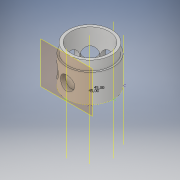
# Autodesk Inventor part: nozzle
Saved by Autodesk Inventor 2019 (Build 230136000, 136)
## iProperties
Created: 2020-10-28
Part Number: nozzle
Material: Genérico
Document SubType Name: Modeling
Designer: Juan M. Casillas
Density: 1 g/cm^3
Appearance: Valor por defecto
Author: Juan M. Casillas
## iProperties of the stored document nozzle_3DPrint.ipt
Created: 2020-10-28
Part Number: nozzle_3DPrint
Material: Genérico
Document SubType Name: Modeling
Designer: Juan M. Casillas
Density: 1 g/cm^3
Appearance: Valor por defecto
Author: Juan M. Casillas
Autodesk Inventor part; units mm, degrees
ref_plane "YZ Plane" through (0, 0, 0) normal (1, 0, 0) x (0, 1, 0)
ref_plane "XZ Plane" through (0, 0, 0) normal (0, 1, 0) x (-1, 0, 0)
ref_plane "XY Plane" through (0, 0, 0) normal (0, 0, 1) x (1, 0, 0)
sketch "Sketch1" plane through (0, 0, 0) normal (0, 1, 0) x (-1, 0, 0)
  circle A0 centre (0, 0) radius 4.65
  circle A1 centre (0, 0) radius 4.05
  dimension "d0" = 9.3
  dimension "d1" = 0.6
  constraints: 2 centre point, 1 coincident
  measures "d0" diameter of A0
  measures "d1" radial gap between concentric circles of A0 A1
extrude "Extrusion1" add sketch "Sketch1" along normal blind 2
sketch "Sketch2" plane through (0, 0, 0) normal (0, -1, 0) x (1, 0, 0)
  circle A0 centre (0, 0) radius 5
  dimension "d4" = 10
  constraints: 1 centre point, 1 coincident
  measures "d4" diameter of A0
extrude "Extrusion2" add sketch "Sketch2" along normal blind 5
sketch "Sketch3" plane through (0, 0, 0) normal (0, 1, 0) x (1, 0, 0)
  circle A0 centre (0, 0) radius 4.05 projected
extrude "Extrusion3" cut sketch "Sketch3" against normal blind 5
sketch "Sketch4" plane through (0, -5, 0) normal (0, -1, 0) x (1, 0, 0)
  circle A0 centre (0, 0) radius 5 projected
extrude "Extrusion4" add sketch "Sketch4" along normal blind 1
sketch "Sketch5" plane through (0, -6, 0) normal (0, -1, 0) x (1, 0, 0)
  line L0 (1, -3) -> (1, 3) construction
  line L1 (-7, 0) -> (7, 0) construction
  circle A0 centre (0, 0) radius 5 construction
  arc A1 (1, -3.873) -> (1, 3.873) centre (0, 0) ccw
  line L2 (1, -3.873) -> (1, 3.873)
  point P0 (1, 0)
  dimension "d11" = 6
  dimension "d12" = 6
  dimension "d13" = 1
  constraints: 4 end point, 2 point on circle, 2 point on line, 1 centre point, 1 midpoint, 1 vertical
  measures "d11" distance of L0.start L0.end
  measures "d13" radial gap between concentric circles of A0 A1
extrude "Extrusion5" cut sketch "Sketch5" against normal blind 1
fillet "Fillet1" radius 0.5 1 edges at (1, -5.5, -3.873)
fillet "Fillet2" radius 0.5 1 edges at (1, -5.5, 3.873)
sketch "Sketch6" plane through (0, -6, 0) normal (0, -1, 0) x (1, 0, 0)
  circle A0 centre (0, 0) radius 5 construction
  line L0 (0, 5) -> (0, -5) construction
  line L1 (5, 0) -> (0, 0) construction
  line L2 (0, 0) -> (3.5355, 3.5355) construction
  line L3 (0, 0) -> (3.5355, -3.5355) construction
  line L4 (0, 0) -> (5, 0) construction
  dimension "d18" = 45
  dimension "d19" = 45
  constraints: 10 end point, 6 point on circle, 4 coincident, 1 equal length, 1 horizontal, 1 perpendicular, 1 vertical
  measures "d18" angle of L1 L2
  measures "d19" angle of L3 L4
ref_plane "Work Plane1" through (0, -6, 5) normal (0, 0, 1) x (1, 0, 0)
sketch "Sketch7" plane through (0, -6, 5) normal (0, 0, 1) x (1, 0, 0)
  circle A0 centre (0, 3) radius 1.5
  line L0 (-5, 0) -> (5, 0) projected
  point P0 (0, 6)
  dimension "d20" = 3
  dimension "d21" = 3
  constraints: 1 centre point
  measures "d20" diameter of A0
  measures "d21" distance from line of L0 A0.centre
extrude "Extrusion6" cut sketch "Sketch7" against normal blind 1.3
pattern_circular "Circular Pattern1" count 5 over 180 about axis through (0, -6, 0) along (0, -1, 0) of "Extrusion6"
body "Solid1"
